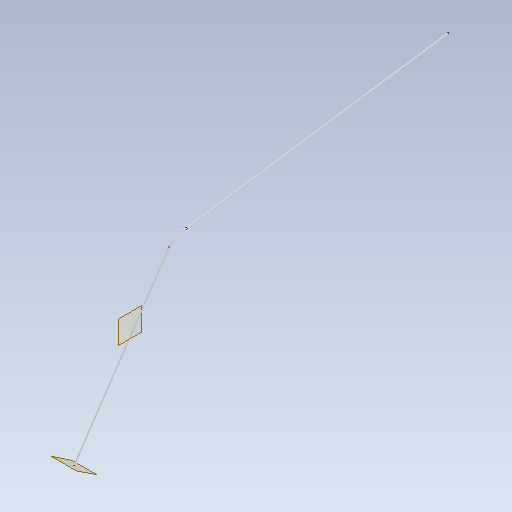
# Autodesk Inventor part: rope
Saved by Autodesk Inventor 2025.2 (Build 292293000, 293)
## iProperties
Created: 2025-03-07
Part Number: rope
Material: Generic
Document SubType Name: Modeling
Designer: email
Density: 1 g/cm^3
Appearance: Default
Author: email
Autodesk Inventor part; units mm, degrees
ref_plane "XZ Plane" through (0, 0, 0) normal (0, 1, 0) x (-1, 0, 0)
ref_plane "XY Plane" through (0, 0, 0) normal (0, 0, 1) x (1, 0, 0)
ref_plane "Work Plane1" through (-31.75, 0, 0) normal (1, 0, 0) x (0, 1, 0)
sketch "Sketch1" plane through (-31.75, 0, 0) normal (1, 0, 0) x (0, 1, 0)
  ellipse E0 centre (-74.6025, 41.3793) end of major axis (-67.6964, 33.1085) minor radius 0.5425 projected
  ellipse E1 centre (-79.5472, 37.2504) end of major axis (-72.641, 28.9797) minor radius 0.5425 projected
  ellipse E2 centre (33.6997, -46.4835) end of major axis (18.5131, -47.1208) minor radius 15.1999 projected
  ellipse E3 centre (56.8416, -277.571) end of major axis (81.8197, -276.5228) minor radius 24.9998 projected
  line L0 (-81.0956, 48.8158) -> (42.1667, -33.8602)
  arc A0 (48.7092, -48.8828) -> (42.1667, -33.8602) centre (33.6998, -46.4835) ccw
  line L1 (48.7092, -48.8828) -> (81.8197, -276.5228)
  point P0 (0, 0)
  constraints: 4 end point, 2 point on circle, 1 centre point, 1 tangent, 8 other
ref_plane "Work Plane2" through (-31.75, -81.0956, 48.8158) normal (0, 0.8305, -0.557) x (-1, 0, 0)
sketch "Sketch2" plane through (-31.75, -81.0956, 48.8158) normal (0, 0.8305, -0.557) x (-1, 0, 0)
  circle A0 centre (0, 0) radius 0.635
  point P0 (-31.75, 4.6322)
  dimension "d11" = 1.27
  constraints: 1 centre point
  measures "d11" diameter of A0
sweep "Sweep1" add profiles "Sketch2" path "Sketch1" path curves L0 A0 L1
body "Solid2"
